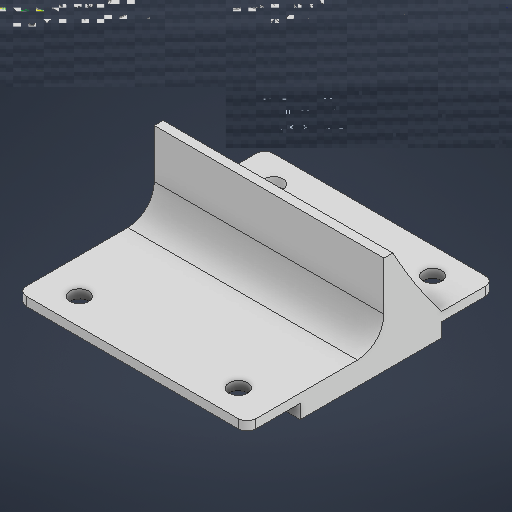
# Autodesk Inventor part: Деталь2
Saved by Autodesk Inventor 2026 (Build 300175000, 175)
## iProperties
Created: 2025-12-24
Part Number: Деталь2
Material: Типовые
Document SubType Name: Modeling
Designer: Phantom_HP2
Density: 1 g/cm^3
Appearance: По умолчанию
Author: Phantom_HP2
Autodesk Inventor part; units mm, degrees
ref_plane "YZ Plane" through (0, 0, 0) normal (1, 0, 0) x (0, 1, 0)
ref_plane "XZ Plane" through (0, 0, 0) normal (0, 1, 0) x (-1, 0, 0)
ref_plane "XY Plane" through (0, 0, 0) normal (0, 0, 1) x (1, 0, 0)
sketch "Эскиз1" plane through (0, 0, 0) normal (0, 1, 0) x (-1, 0, 0)
  line L0 (0, 0) -> (52, 0)
  line L1 (52, 0) -> (52, -56)
  line L2 (52, -56) -> (0, -56)
  line L3 (0, -56) -> (0, 0)
  dimension "d0" = 56
  dimension "d9" = 52
  constraints: 8 end point, 2 parallel, 1 horizontal, 1 perpendicular
  measures "d0" distance of L0.end L1.end
  measures "d9" distance of L1.end L2.end
extrude "Выдавливание1" add sketch "Эскиз1" along normal blind 5.2
sketch "Эскиз2" plane through (0, 0, 0) normal (1, 0, 0) x (0, 0, -1)
  line L0 (56, 0) -> (0, 0) projected
  line L1 (0, 0) -> (12, 0)
  line L2 (12, 0) -> (12, 3.2)
  line L3 (12, 3.2) -> (0, 3.2)
  line L4 (0, 3.2) -> (0, 0)
  line L5 (56, 0) -> (56, 5.2) projected
  line L6 (56, 0) -> (44, 0)
  line L7 (44, 0) -> (44, 3.2)
  line L8 (44, 3.2) -> (56, 3.2)
  line L9 (56, 3.2) -> (56, 0)
  dimension "d3" = 12
  dimension "d4" = 3.2
  dimension "d5" = 12
  dimension "d6" = 3.2
  constraints: 16 end point, 4 parallel, 2 horizontal, 2 perpendicular
  measures "d3" distance of L3.end L2.end
  measures "d4" distance of L1.end L2.end
  measures "d5" distance of L7.end L8.end
  measures "d6" distance of L6.end L7.end
extrude "Выдавливание2" cut sketch "Эскиз2" against normal up to surface (52 mm away)
sketch "Эскиз3" plane through (0, 3.2, -12) normal (0, -1, 0) x (1, 0, 0)
  circle A0 centre (-8, 6) radius 2.1
  line L0 (0, 12) -> (0, 0) projected
  line L1 (-52, 12) -> (0, 12) projected
  circle A1 centre (-44, 6) radius 2.1
  line L2 (-52, 0) -> (-52, 12) projected
  circle A2 centre (-44, -38) radius 2.1
  line L3 (-52, -44) -> (-52, -32) projected
  line L4 (0, -44) -> (-52, -44) projected
  circle A3 centre (-8, -38) radius 2.1
  line L5 (0, -32) -> (0, -44) projected
  point P0 (0, 6)
  dimension "d10" = 4.2
  dimension "d11" = 8
  dimension "d12" = 6
  dimension "d13" = 4.2
  dimension "d14" = 6
  dimension "d15" = 8
  dimension "d16" = 4.2
  dimension "d17" = 8
  dimension "d18" = 6
  dimension "d19" = 4.2
  dimension "d20" = 8
  dimension "d21" = 6
  constraints: 4 centre point, 1 midpoint
  measures "d10" diameter of A0
  measures "d11" distance of point (0, 6) A0.centre
  measures "d12" distance from line of L1 A0.centre
  measures "d13" diameter of A1
  measures "d14" distance from line of L1 A1.centre
  measures "d15" distance from line of L2 A1.centre
  measures "d16" diameter of A2
  measures "d17" distance from line of L3 A2.centre
  measures "d18" distance from line of L4 A2.centre
  measures "d19" diameter of A3
  measures "d20" distance from line of L5 A3.centre
  measures "d21" distance from line of L4 A3.centre
extrude "Выдавливание3" cut sketch "Эскиз3" against normal blind 10
fillet "Сопряжение1" radius 2 4 edges at (0, 4.2, 0) (0, 4.2, -56) (-52, 4.2, -56) (-52, 4.2, 0)
sketch "Эскиз4" plane through (0, 0, -12) normal (1, 0, 0) x (0, 0, -1)
  line L0 (31.9749, 5.2) -> (18.9749, 5.2)
  line L1 (18.9749, 22.2) -> (18.9749, 5.2)
  line L2 (18.9749, 22.2) -> (20.9749, 22.2)
  arc A0 (20.9749, 22.2) -> (31.9749, 5.2) centre (135.2876, 84.1082) ccw
  point P0 (-12, 0)
  dimension "d26" = 13
  dimension "d34" = 2
  dimension "d35" = 130
  constraints: 6 end point, 2 point on circle, 1 centre point, 1 horizontal
  measures "d26" distance of L0.start L0.end
  measures "d34" distance of L1.start L2.end
  measures "d35" radius of A0
extrude "Выдавливание4" add sketch "Эскиз4" against normal up to surface (52 mm away)
fillet "Сопряжение3" radius 6 1 edges at (-26, 5.2, -30.9749)
